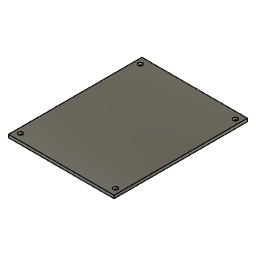
Back Panel (Autodesk Fusion 360 design; units mm, degrees)
Autodesk Fusion 360 part; units mm, degrees
sketch "Sketch1" plane through (0, 0, 0) normal (0, 0, 1) x (1, 0, 0)
  line L0 (0, 0) -> (70.25, 0)
  line L1 (70.25, 0) -> (70.25, 88.75)
  line L2 (70.25, 88.75) -> (0, 88.75)
  line L3 (0, 88.75) -> (0, 0)
  point P0 (3.5, 84.25)
  point P1 (66.75, 84.25)
  point P2 (3.5, 4.5)
  point P3 (66.75, 4.5)
  dimension "d1" = 88.75
  dimension "d2" = 70.25
  dimension "d8" = 3.5
  dimension "d9" = 4.5
  dimension "d10" = 3.5
  dimension "d11" = 4.5
  dimension "d12" = 3.5
  dimension "d13" = 4.5
  dimension "d14" = 4.5
  dimension "d15" = 3.5
  constraint horizontal L0
  constraint vertical L1
  constraint horizontal L2
  constraint vertical L3
  constraint coincident L0.start L3.end
  measures "d1" distance of L0.start L2.end
  measures "d2" distance of L0.start L0.end
  measures "d8" distance of L3 P0
  measures "d9" distance of L2 P0
  measures "d10" distance of L1 P1
  measures "d11" distance of L2 P1
  measures "d12" distance of L3 P2
  measures "d13" distance of L0 P2
  measures "d14" distance of L0 P3
  measures "d15" distance of L1 P3
extrude "Extrude1" add sketch "Sketch1" against normal blind 2
hole "Hole1" at (66.75, 84.25, 0) at (3.5, 84.25, 0) at (66.75, 4.5, 0) at (3.5, 4.5, 0) direction (0, 0, -1) diameter 1.5 end through all countersink diameter 3 countersink angle 82
